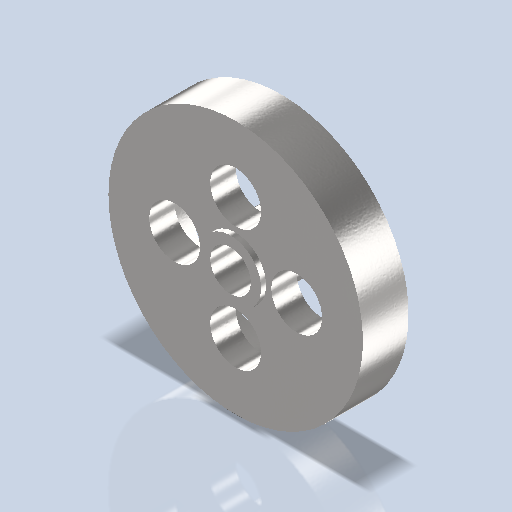
# Autodesk Inventor part: Schwungscheibe
Saved by Autodesk Inventor 2024 (Build 280153000, 153)
## iProperties
Created: 2024-01-15
Part Number: Schwungscheibe
Material: Stahl, galvanisiert
Document SubType Name: Modeling
Designer: ffogue
Density: 7.85 g/cm^3
Appearance: Galvanisiert
Author: ffogue
Autodesk Inventor part; units mm, degrees
ref_plane "YZ Plane" through (0, 0, 0) normal (1, 0, 0) x (0, 1, 0)
ref_plane "XZ Plane" through (0, 0, 0) normal (0, 1, 0) x (-1, 0, 0)
ref_plane "XY Plane" through (0, 0, 0) normal (0, 0, 1) x (1, 0, 0)
sketch "Skizze4" plane through (0, 0, 0) normal (0, 0, 1) x (1, 0, 0)
  line L0 (25, 9) -> (25, -1)
  line L1 (25, 9) -> (7, 9)
  line L2 (12.1242, 0) -> (0, 0)
  line L3 (0, 0) -> (0, 9)
  line L4 (0, 9) -> (7, 9)
  line L5 (9.9688, 0) -> (19, 0)
  line L6 (19, 0) -> (19, -1)
  line L7 (19, -1) -> (25, -1)
  point P0 (6.0621, 0)
  dimension "d6" = 50
  dimension "d7" = 1
  dimension "d8" = 10
  dimension "d11" = 12
  constraints: 16 end point, 3 perpendicular, 3 point on line, 1 coincident, 1 horizontal, 1 midpoint, 1 vertical
  measures "d6" diameter of L3 L0
  measures "d7" distance from line of L7 point (6.062, 0)
  measures "d8" distance between parallel lines of L7 L4
  measures "d11" diameter of L6 L0
revolve "Umdrehung1" add sketch "Skizze4" angle 360 about axis through (25, 9, 0) along (0, -1, 0)
sketch "Skizze5" plane through (25, 9, 0) normal (0, 1, 0) x (1, 0, 0)
  circle A0 centre (0, 0) radius 6 projected
  circle A1 centre (0, 0) radius 18
  point P0 (-25, 0)
  dimension "d20" = 36
  constraints: 1 centre point, 1 coincident
  measures "d20" diameter of A1
extrude "Extrusion3" cut sketch "Skizze5" against normal blind 4
sketch "Skizze6" plane through (25, 9, 0) normal (0, 1, 0) x (1, 0, 0)
  circle A0 centre (0, 0) radius 6 projected
  point P0 (-25, 0)
  constraints: 1 coincident
hole "Bohrung1" at (25, 9, 0) direction (0, -1, 0) diameter 8 end through all
sketch "Skizze7" plane through (25, 0, 0) normal (0, -1, 0) x (1, 0, 0)
  circle A0 centre (0, 0) radius 4 projected
  line L0 (0, 2.1422) -> (0, -2.7169) construction
  point P0 (-25, 0)
  point P1 (12, 0)
  point P2 (-12, 0)
  dimension "d31" = 24
  constraints: 2 end point, 2 horizontal alignment, 1 symmetric about line, 1 vertical
  measures "d31" distance of point (12, 0) point (-12, 0)
hole "Bohrung2" at (37, 0, 0) at (13, 0, 0) direction (0, 1, 0) diameter 10 end through all
pattern_circular "Runde Anordnung1" count 4 over 360 about axis through (25, 4.5, 0) along (0, -1, 0) of "Bohrung2"
